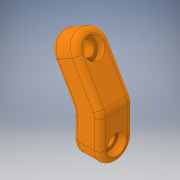
# Autodesk Inventor part: Link2
Saved by Autodesk Inventor 2019 (Build 230136000, 136)
## iProperties
Created: 2022-07-14
Part Number: Link2
Material: Generic
Document SubType Name: Modeling
Designer: zreik
Density: 1 g/cm^3
Appearance: Orange
d46: 10.000 mm
Author: zreik
Autodesk Inventor part; units mm, degrees
ref_plane "YZ Plane" through (0, 0, 0) normal (1, 0, 0) x (0, 1, 0)
sketch "Sketch1" plane through (0, 0, 0) normal (0, 0, 1) x (1, 0, 0)
  line L0 (53.588457, 0) -> (0, 0)
  line L1 (0, 0) -> (60.328682, 34.830781)
  line L2 (43.588457, 0) -> (43.588457, 7.660254)
  line L3 (42.918584, 10.160254) -> (36.588457, 21.124356)
  line L4 (53.588457, 0) -> (53.588457, 10.339746)
  line L5 (52.918584, 12.839746) -> (45.248711, 26.124356)
  arc A0 (43.588457, 7.660254) -> (42.918584, 10.160254) centre (38.588457, 7.660254) ccw
  arc A1 (53.588457, 10.339746) -> (52.918584, 12.839746) centre (48.588457, 10.339746) ccw
  line L6 (45.248711, 26.124356) -> (36.588457, 21.124356)
  line L7 (45.248711, 26.124356) -> (52.918584, 12.839746)
  line L8 (36.588457, 21.124356) -> (42.918584, 10.160254)
  line L9 (43.588457, 0) -> (53.588457, 0)
  line L10 (53.588457, 0) -> (53.588457, 10.339746)
  line L11 (43.588457, 0) -> (53.588457, 0)
  line L12 (53.588457, 0) -> (53.588457, 10.339746)
  line L13 (52.918584, 12.839746) -> (45.248711, 26.124356)
  line L14 (45.248711, 26.124356) -> (36.588457, 21.124356)
  line L15 (36.588457, 21.124356) -> (42.918584, 10.160254)
  line L16 (43.588457, 7.660254) -> (43.588457, 0)
  point P0 (43.30127, 25)
  point P1 (43.588457, 9)
  dimension "d37" = 30
  dimension "d38" = 10
  dimension "d39" = 10
  dimension "d40" = 0
  dimension "d41" = 0
  dimension "d42" = 9
  dimension "d43" = 14
  dimension "d44" = 150
  dimension "d45" = 5
  constraints: 34 end point, 9 collinear, 6 point on line, 4 point on circle, 4 tangent, 2 centre point, 2 parallel, 1 coincident, 1 equal radius, 1 horizontal, 1 vertical
  measures "d37" angle of L1 L0
  measures "d38" distance between parallel lines of L3 L5
  measures "d39" distance between parallel lines of L4 L2
  measures "d40" distance from line of L1 L3.end
  measures "d41" distance from line of L1 L5.end
  measures "d42" distance of L2.start point (43.588, 9)
  measures "d43" distance of point (43.588, 9) L3.end
  measures "d44" angle of L2 L3
  measures "d45" radius of A0
extrude "Extrusion1" add sketch "Sketch1" along normal blind 12 contours L0 L2 A0 L3 L1 L5 A1 L4
ref_plane "Work Plane1" through (52.918584, 12.839746, 0) normal (0.8660254, 0.5, 0) x (-0.5, 0.8660254, 0)
sketch "Sketch2" plane through (52.918584, 12.839746, 0) normal (0.8660254, 0.5, 0) x (-0.5, 0.8660254, 0)
  circle A0 centre (15.339746, 6) radius 6
  line L0 (15.339746, 0) -> (15.339746, 12)
  line L1 (0, 12) -> (15.339746, 12)
  dimension "d5" = 12
  dimension "d47" = 0
  dimension "d48" = 6
  constraints: 1 centre point
  measures "d5" diameter of A0
  measures "d47" distance from line of L0 A0.centre
  measures "d48" distance from line of L1 A0.centre
extrude "Extrusion2" add sketch "Sketch2" against normal blind 10
ref_plane "Work Plane2" through (53.588457, 10.339746, 0) normal (1, 0, 0) x (0, 1, 0)
sketch "Sketch3" plane through (53.588457, 10.339746, 0) normal (1, 0, 0) x (0, 1, 0)
  circle A0 centre (-10.339746, 6) radius 6
  line L0 (-10.339746, 0) -> (-10.339746, 12)
  line L1 (-10.339746, 0) -> (0, 0)
  point P0 (43.30127, 10)
  point P1 (10.78461, 12)
  dimension "d10" = 12
  dimension "d49" = 0
  dimension "d50" = 6
  constraints: 1 centre point, 1 other
  measures "d10" diameter of A0
  measures "d49" distance from line of L0 A0.centre
  measures "d50" distance from line of L1 A0.centre
extrude "Extrusion3" add sketch "Sketch3" against normal blind 10
sketch "Sketch4" plane through (44.25833, 7.839746, 0) normal (-0.8660254, -0.5, 0) x (0.5, -0.8660254, 0)
  circle A0 centre (-15.339746, 6) radius 2.5
  circle A1 centre (-15.339746, 6) radius 6
  point P0 (-15.339746, 0)
  point P1 (-15.339746, 12)
  dimension "d15" = 5
  constraints: 1 centre point, 1 concentric
  measures "d15" diameter of A0
extrude "Extrusion4" cut sketch "Sketch4" along normal through all both and the other way through all contours A0
sketch "Sketch5" plane through (43.588457, 10.339746, 0) normal (-1, 0, 0) x (0, 0, 1)
  circle A0 centre (6, -10.339746) radius 2.5
  arc A1 (0, -10.339746) -> (12, -10.339746) centre (6, -10.339746) ccw
  dimension "d18" = 5
  constraints: 1 centre point, 1 concentric
  measures "d18" diameter of A0
extrude "Extrusion5" cut sketch "Sketch5" along normal through all both and the other way through all
sketch "Sketch6" plane through (52.918584, 12.839746, 0) normal (0.8660254, 0.5, 0) x (0.5, -0.8660254, 0)
  circle A0 centre (-15.339746, -6) radius 3.6
  circle A1 centre (-15.339746, -6) radius 2.5
  arc A2 (-15.339746, 0) -> (-15.339746, 0) centre (-15.339746, -6) ccw
  point P0 (0, -10)
  dimension "d21" = 5
  dimension "d22" = 7.2
  constraints: 2 centre point, 1 coincident, 2 other
  measures "d21" diameter of A1
  measures "d22" diameter of A0
extrude "Extrusion6" cut sketch "Sketch6" against normal blind 3 contours A0
sketch "Sketch7" plane through (44.25833, 7.839746, 0) normal (-0.8660254, -0.5, 0) x (0.5, -0.8660254, 0)
  circle A0 centre (-15.339746, 6) radius 3.6
  circle A1 centre (-15.339746, 6) radius 2.5
  arc A2 (-12.839746, 6) -> (-12.839746, 6) centre (-15.339746, 6) ccw
  point P0 (-15.339746, 0)
  dimension "d25" = 5
  dimension "d26" = 7.2
  constraints: 2 centre point, 1 coincident, 1 concentric
  measures "d25" diameter of A1
  measures "d26" diameter of A0
extrude "Extrusion7" cut sketch "Sketch7" along normal mid plane 6
sketch "Sketch8" plane through (43.588457, 10.339746, 0) normal (-1, 0, 0) x (0, 0, 1)
  circle A0 centre (6, -10.339746) radius 3.6
  circle A1 centre (6, -10.339746) radius 2.5
  arc A2 (8.5, -10.339746) -> (8.5, -10.339746) centre (6, -10.339746) ccw
  point P0 (0, -10.339746)
  dimension "d29" = 7.2
  dimension "d30" = 5
  constraints: 2 centre point, 1 coincident, 1 concentric
  measures "d29" diameter of A0
  measures "d30" diameter of A1
extrude "Extrusion8" cut sketch "Sketch8" along normal mid plane 6
sketch "Sketch9" plane through (53.588457, 10.339746, 0) normal (1, 0, 0) x (0, 0, -1)
  circle A0 centre (-6, -10.339746) radius 3.6
  circle A1 centre (-6, -10.339746) radius 2.5
  circle A2 centre (-6, -10.339746) radius 2.5
  point P0 (0, -10.339746)
  dimension "d33" = 5
  dimension "d34" = 7.2
  constraints: 2 centre point, 1 coincident, 1 concentric
  measures "d33" diameter of A1
  measures "d34" diameter of A0
extrude "Extrusion9" cut sketch "Sketch9" against normal blind 3
fillet "Fillet1" radius 2 16 edges at (42.2487, 31.3205, 6) (49.0836, 19.4821, 0) (53.4181, 11.6338, 0) (53.5885, 5.1699, 0) (53.5885, -6, 6) (53.5885, 5.1699, 12) (53.4181, 11.6338, 12) (49.0836, 19.4821, 12) (43.4181, 8.9543, 12) (43.5885, 3.8301, 12) (43.5885, -6, 6) (43.5885, 3.8301, 0) (43.4181, 8.9543, 0) (39.7535, 15.6423, 0) (33.5885, 26.3205, 6) (39.7535, 15.6423, 12)
equation "\"d38\" = d46"
equation "\"d39\" = d46"
equation "\"d3\" = width"
equation "\"d5\" = width"
equation "\"d48\" = 0.5 * width"
equation "\"d8\" = thickness"
equation "\"d10\" = width"
equation "\"d50\" = 0.5 * width"
equation "\"d13\" = thickness"
equation "\"thickness\" = 10"
equation "\"width\" = 12"
equation "\"d46\" = 10"
body "Solid1"
